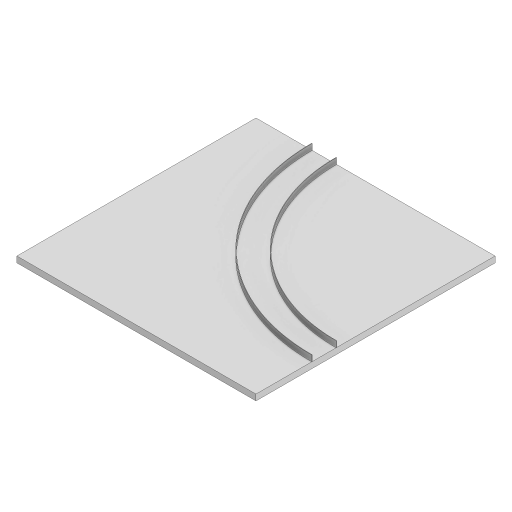
# Autodesk Inventor part: curve
Saved by Autodesk Inventor 2023 (Build 270158000, 158)
## iProperties
Created: 2022-07-11
Part Number: curve
Material: Generic
Document SubType Name: Modeling
Designer: Derm
Density: 1 g/cm^3
Appearance: Default
Author: Derm
Autodesk Inventor part; units mm, degrees
ref_plane "YZ Plane" through (0, 0, 0) normal (1, 0, 0) x (0, 1, 0)
ref_plane "XZ Plane" through (0, 0, 0) normal (0, 1, 0) x (-1, 0, 0)
ref_plane "XY Plane" through (0, 0, 0) normal (0, 0, 1) x (1, 0, 0)
sketch "Sketch1" plane through (0, 0, 0) normal (0, 1, 0) x (-1, 0, 0)
  line L0 (-50000, 50000) -> (50000, 50000)
  line L1 (50000, 50000) -> (50000, -50000)
  line L2 (50000, -50000) -> (-50000, -50000)
  line L3 (-50000, -50000) -> (-50000, 50000)
  line L4 (-50000, 50000) -> (50000, -50000) construction
  line L5 (50000, 50000) -> (-50000, -50000) construction
  point P0 (0, 0)
  dimension "d0" = 100000
  dimension "d1" = 100000
  constraints: 12 end point, 2 midpoint, 2 parallel, 1 horizontal, 1 perpendicular
  measures "d0" distance of L0.end L1.end
  measures "d1" distance of L1.end L2.end
extrude "Extrusion1" add sketch "Sketch1" against normal blind 2500
sketch "Sketch2" plane through (0, 0, 0) normal (0, 1, 0) x (1, 0, 0)
  line L0 (-50000, 50000) -> (50000, 50000) projected
  line L1 (50000, 50000) -> (50000, -50000) projected
  arc A0 (0, 50000) -> (50000, 0) centre (50000, 50000) ccw construction
  arc A1 (-26506.6822, 50000) -> (50000, -26506.6822) centre (50000, 50000) ccw
  arc A2 (-16506.6822, 50000) -> (50000, -16506.6822) centre (50000, 50000) ccw
  arc A3 (-26709.8822, 50000) -> (50000, -26709.8822) centre (50000, 50000) ccw
  arc A4 (-16303.4822, 50000) -> (50000, -16303.4822) centre (50000, 50000) ccw
  point P0 (0, 0)
  point P1 (50000, -16303.4822)
  point P2 (50000, -26709.8822)
  dimension "d5" = 203.2
  dimension "d6" = 203.2
  dimension "d7" = 10000
  constraints: 10 point on circle, 5 centre point, 2 midpoint, 2 point on line
  measures "d5" radial gap between concentric circles of A3 A1
  measures "d6" radial gap between concentric circles of A4 A2
  measures "d7" radial gap between concentric circles of A2 A1
extrude "Extrusion2" add sketch "Sketch2" along normal blind 2500 contours L0 A1 L1 A3 | L0 A4 L1 A2
body "Solid1"
